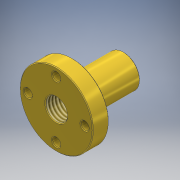
# Autodesk Inventor part: Tin-bronze M8 nut for Z- axis
Saved by Autodesk Inventor 2016 (Build 200138000, 138)
## iProperties
Created: 2016-04-10
Part Number: Tin-bronze M8 nut for Z- axis
Material: Типовые
Document SubType Name: Modeling
Designer: Admin
Density: 1 g/cm^3
Appearance: По умолчанию
Author: Admin
Autodesk Inventor part; units mm, degrees
ref_plane "YZ Plane" through (0, 0, 0) normal (1, 0, 0) x (0, 1, 0)
ref_plane "XZ Plane" through (0, 0, 0) normal (0, 1, 0) x (-1, 0, 0)
ref_plane "XY Plane" through (0, 0, 0) normal (0, 0, 1) x (1, 0, 0)
sketch "Эскиз1" plane through (0, 0, 0) normal (0, 1, 0) x (-1, 0, 0)
  circle A0 centre (0, 0) radius 13.5
  dimension "d0" = 27
  constraints: 1 centre point, 1 coincident
  measures "d0" diameter of A0
extrude "Выдавливание1" add sketch "Эскиз1" along normal blind 6
sketch "Эскиз2" plane through (0, 6, 0) normal (0, 1, 0) x (1, 0, 0)
  circle A0 centre (0, 0) radius 6
  dimension "d3" = 12
  constraints: 1 centre point, 1 coincident
  measures "d3" diameter of A0
extrude "Выдавливание2" add sketch "Эскиз2" along normal blind 19
sketch "Эскиз3" plane through (0, 25, 0) normal (0, 1, 0) x (1, 0, 0)
  circle A0 centre (0, 0) radius 4
  dimension "d6" = 8
  constraints: 1 centre point, 1 coincident
  measures "d6" diameter of A0
extrude "Выдавливание3" cut sketch "Эскиз3" against normal through all
chamfer "Фаска1" distance 0.25 angle 45 5 edges at (-4, 25, 0) (-6, 25, 0) (13.5, 6, 0) (13.5, 0, 0) (-4, 0, 0)
sketch "Эскиз4" plane through (0, 6, 0) normal (0, 1, 0) x (1, 0, 0)
  circle A0 centre (0, -10.5) radius 1.5
  circle A1 centre (-10.5, 0) radius 1.5
  circle A2 centre (0, 10.5) radius 1.5
  circle A3 centre (10.5, 0) radius 1.5
  dimension "d13" = 3
  dimension "d14" = 3
  dimension "d15" = 3
  dimension "d16" = 3
  constraints: 4 centre point
  measures "d13" diameter of A0
  measures "d14" diameter of A1
  measures "d15" diameter of A2
  measures "d16" diameter of A3
extrude "Выдавливание4" cut sketch "Эскиз4" against normal through all
chamfer "Фаска2" distance 0.25 angle 45 8 edges at (-12, 6, 0) (-1.5, 6, -10.5) (9, 6, 0) (-1.5, 6, 10.5) (-1.5, 0, 10.5) (-12, 0, 0) (9, 0, 0) (-1.5, 0, -10.5)
thread "Резьба1" size "M8x1.25" class "6H" standard "ANSI Metric M Profile" full length
